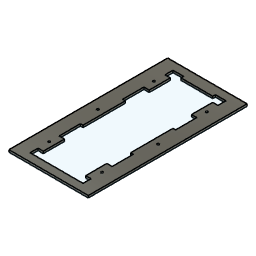
Potoboard holder v5 (Autodesk Fusion 360 design; units mm, degrees)
Autodesk Fusion 360 part; units mm, degrees
sketch "Sketch1" plane through (0, 0, 0) normal (0, 0, 1) x (1, 0, 0)
  line L0 (-75, 150) -> (75, 150)
  line L1 (75, 150) -> (75, -150)
  line L2 (75, -150) -> (-75, -150)
  line L3 (-75, -150) -> (-75, 150)
  line L4 (-75, 150) -> (75, -150) construction
  line L5 (75, 150) -> (-75, -150) construction
  line L6 (50, 135) -> (-50, 135)
  line L7 (-50, 135) -> (-50, -135)
  line L8 (-50, -135) -> (50, -135)
  line L9 (50, -135) -> (50, 135)
  line L10 (50, 135) -> (-50, -135) construction
  line L11 (-50, 135) -> (50, -135) construction
  line L12 (-30, 135) -> (30, 135)
  line L13 (30, 135) -> (30, 130)
  line L14 (30, 130) -> (-30, 130)
  line L15 (-30, 130) -> (-30, 135)
  line L16 (-50, 40) -> (-45, 40)
  line L17 (-45, 40) -> (-45, -40)
  line L18 (-45, -40) -> (-50, -40)
  line L19 (-50, -40) -> (-50, 40)
  line L20 (-30, -135) -> (30, -135)
  line L21 (30, -135) -> (30, -130)
  line L22 (30, -130) -> (-30, -130)
  line L23 (-30, -130) -> (-30, -135)
  line L24 (50, 40) -> (45, 40)
  line L25 (45, 40) -> (45, -40)
  line L26 (45, -40) -> (50, -40)
  line L27 (50, -40) -> (50, 40)
  line L28 (-50, -80) -> (-40, -80)
  line L29 (-40, -80) -> (-40, -120)
  line L30 (-40, -120) -> (-50, -120)
  line L31 (-50, -120) -> (-50, -80)
  line L32 (50, -120) -> (40, -120)
  line L33 (40, -120) -> (40, -80)
  line L34 (40, -80) -> (50, -80)
  line L35 (50, -80) -> (50, -120)
  line L36 (50, 120) -> (40, 120)
  line L37 (40, 120) -> (40, 80)
  line L38 (40, 80) -> (50, 80)
  line L39 (50, 80) -> (50, 120)
  line L40 (-50, 120) -> (-40, 120)
  line L41 (-40, 120) -> (-40, 80)
  line L42 (-40, 80) -> (-50, 80)
  line L43 (-50, 80) -> (-50, 120)
  dimension "d1" = 300
  dimension "d2" = 150
  dimension "d3" = 270
  dimension "d4" = 100
  dimension "d5" = 60
  dimension "d6" = 20
  dimension "d7" = 5
  dimension "d8" = 80
  dimension "d9" = 95
  dimension "d10" = 5
  dimension "d11" = 60
  dimension "d12" = 5
  dimension "d13" = 20
  dimension "d14" = 80
  dimension "d15" = 5
  dimension "d16" = 95
  dimension "d19" = 10
  dimension "d20" = 40
  dimension "d21" = 40
  dimension "d22" = 10
  dimension "d23" = 40
  dimension "d24" = 40
  dimension "d25" = 10
  dimension "d26" = 40
  dimension "d27" = 40
  dimension "d28" = 10
  dimension "d29" = 40
  dimension "d30" = 40
  constraint horizontal L0
  constraint perpendicular L0 L1
  constraint parallel L0 L2
  constraint parallel L1 L3
  constraint coincident L4 origin
  constraint coincident L5 origin
  constraint horizontal L6
  constraint perpendicular L6 L7
  constraint parallel L6 L8
  constraint parallel L7 L9
  constraint coincident L10 origin
  constraint coincident L11 origin
  constraint horizontal L12
  constraint vertical L13
  constraint horizontal L14
  constraint vertical L15
  constraint coincident L6 L12.start
  constraint horizontal L16
  constraint vertical L17
  constraint horizontal L18
  constraint vertical L19
  constraint coincident L7 L16.start
  constraint horizontal L20
  constraint vertical L21
  constraint horizontal L22
  constraint vertical L23
  constraint coincident L8 L20.start
  constraint horizontal L24
  constraint vertical L25
  constraint horizontal L26
  constraint vertical L27
  constraint coincident L9 L24.start
  constraint horizontal L28
  constraint vertical L29
  constraint horizontal L30
  constraint vertical L31
  constraint coincident L7 L28.start
  constraint horizontal L32
  constraint vertical L33
  constraint horizontal L34
  constraint vertical L35
  constraint coincident L9 L32.start
  constraint horizontal L36
  constraint vertical L37
  constraint horizontal L38
  constraint vertical L39
  constraint coincident L9 L36.start
  constraint horizontal L40
  constraint vertical L41
  constraint horizontal L42
  constraint vertical L43
  constraint coincident L7 L40.start
  measures "d1" distance of L0.start L2.end
  measures "d2" distance of L0.start L0.end
  measures "d3" distance of L6.end L7.end
  measures "d4" distance of L6.start L6.end
  measures "d5" distance of L13.end L14.end
  measures "d6" distance of L6.end L12.start
  measures "d7" distance of L12.end L13.end
  measures "d8" distance of L16.end L17.end
  measures "d9" distance of L6.end L16.start
  measures "d10" distance of L17.end L18.end
  measures "d11" distance of L21.end L22.end
  measures "d12" distance of L20.start L22.end
  measures "d13" distance of L7.end L20.start
  measures "d14" distance of L24.end L25.end
  measures "d15" distance of L24.start L24.end
  measures "d16" distance of L6.start L24.start
  measures "d19" distance of L28.start L28.end
  measures "d20" distance of L28.end L29.end
  measures "d21" distance of L18.end L28.start
  measures "d22" distance of L32.start L32.end
  measures "d23" distance of L32.end L33.end
  measures "d24" distance of L26.end L34.end
  measures "d25" distance of L36.start L36.end
  measures "d26" distance of L36.end L37.end
  measures "d27" distance of L24 L38.end
  measures "d28" distance of L40.start L40.end
  measures "d29" distance of L40.end L41.end
  measures "d30" distance of L16.start L42.end
extrude "Extrude2" add sketch "Sketch1" along normal blind 4 contours L0 L1 L2 L3 | L6 L12 L13 L14 L15 | L9 L36 L37 L38 L39 | L9 L24 L25 L26 L27 | L7 L40 L41 L42 L43 | L9 L32 L33 L34 L35 | L7 L16 L17 L18 L19 | L7 L28 L29 L30 L31
sketch "Sketch2" plane through (0, 0, 0) normal (0, 0, 1) x (1, 0, 0)
  line L0 (0, 0) -> (-57, 0) construction
  circle A0 centre (-57, 0) radius 2
  line L1 (0, 0) -> (57, 0) construction
  circle A1 centre (57, 0) radius 2
  line L2 (0, 0) -> (0, -99) construction
  line L3 (0, -99) -> (-50, -99) construction
  line L4 (0, -99) -> (50, -99) construction
  line L5 (0, 0) -> (0, 99) construction
  line L6 (0, 99) -> (50, 99) construction
  line L7 (0, 99) -> (-50, 99) construction
  circle A2 centre (50, 99) radius 2
  circle A3 centre (-50, 99) radius 2
  circle A4 centre (50, -99) radius 2
  circle A5 centre (-50, -99) radius 2
  dimension "d33" = 57
  dimension "d35" = 4
  dimension "d36" = 57
  dimension "d37" = 4
  dimension "d38" = 99
  dimension "d39" = 50
  dimension "d40" = 50
  dimension "d41" = 99
  dimension "d42" = 50
  dimension "d43" = 4
  dimension "d44" = 4
  dimension "d45" = 50
  dimension "d46" = 4
  dimension "d47" = 4
  constraint coincident L0.start L1.start
  constraint horizontal L0
  constraint coincident L0.end A0.centre
  constraint parallel L0 L1
  constraint coincident L1.end A1.centre
  constraint perpendicular L1 L2
  constraint perpendicular L2 L3
  constraint perpendicular L2 L4
  constraint perpendicular L0 L5
  constraint perpendicular L5 L6
  constraint perpendicular L5 L7
  constraint coincident L6.end A2.centre
  constraint coincident L7.end A3.centre
  constraint coincident L4.end A4.centre
  constraint coincident L3.end A5.centre
  measures "d33" distance of L0.start L0.end
  measures "d35" diameter of A0
  measures "d36" distance of L0.start L1.end
  measures "d37" diameter of A1
  measures "d38" distance of L0.start L2.end
  measures "d39" distance of L2.end L3.end
  measures "d40" distance of L2.end L4.end
  measures "d41" distance of L0.start L5.end
  measures "d42" distance of L5.end L6.end
  measures "d43" diameter of A2
  measures "d44" diameter of A3
  measures "d45" distance of L5.end L7.end
  measures "d46" diameter of A4
  measures "d47" diameter of A5
extrude "Extrude3" cut sketch "Sketch2" along normal through all
sketch "Sketch3" plane through (0, 0, 0) normal (0, 0, -1) x (1, 0, 0)
  circle A0 centre (57, 0) radius 2
  circle A1 centre (-50, 99) radius 2
  circle A2 centre (-50, -99) radius 2
  circle A3 centre (-57, 0) radius 2
  circle A4 centre (50, 99) radius 2
  circle A5 centre (50, -99) radius 2
  line L0 (50, -120) -> (50, -135)
  line L1 (50, -135) -> (30, -135)
  line L2 (30, -135) -> (30, -130)
  line L3 (30, -130) -> (-30, -130)
  line L4 (-30, -130) -> (-30, -135)
  line L5 (-30, -135) -> (-50, -135)
  line L6 (-50, -135) -> (-50, -120)
  line L7 (-50, -120) -> (-40, -120)
  line L8 (-40, -120) -> (-40, -80)
  line L9 (-40, -80) -> (-50, -80)
  line L10 (-50, -80) -> (-50, -40)
  line L11 (-50, -40) -> (-45, -40)
  line L12 (-45, -40) -> (-45, 40)
  line L13 (-45, 40) -> (-50, 40)
  line L14 (-50, 40) -> (-50, 80)
  line L15 (-50, 80) -> (-40, 80)
  line L16 (-40, 80) -> (-40, 120)
  line L17 (-40, 120) -> (-50, 120)
  line L18 (-50, 120) -> (-50, 135)
  line L19 (-50, 135) -> (50, 135)
  line L20 (50, 135) -> (50, 120)
  line L21 (50, 120) -> (40, 120)
  line L22 (40, 120) -> (40, 80)
  line L23 (40, 80) -> (50, 80)
  line L24 (50, 80) -> (50, 40)
  line L25 (50, 40) -> (45, 40)
  line L26 (45, 40) -> (45, -40)
  line L27 (45, -40) -> (50, -40)
  line L28 (50, -40) -> (50, -80)
  line L29 (50, -80) -> (40, -80)
  line L30 (40, -80) -> (40, -120)
  line L31 (40, -120) -> (50, -120)
  line L32 (75, 150) -> (-75, 150)
  line L33 (-75, 150) -> (-75, -150)
  line L34 (-75, -150) -> (75, -150)
  line L35 (75, -150) -> (75, 150)
